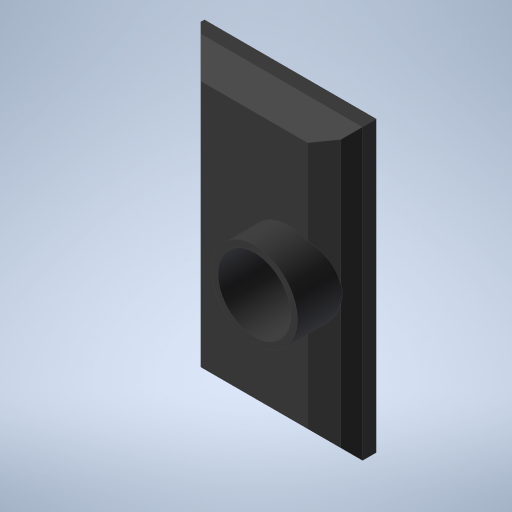
# Autodesk Inventor part: Part5
Saved by Autodesk Inventor 2024 (Build 280153000, 153)
## iProperties
Created: 2024-06-14
Part Number: Part5
Material: Generic
Document SubType Name: Sheet Metal
Designer: albah
Density: 1 g/cm^3
Sheet Metal Rule: Default_mm
Appearance: Default
Author: albah
Autodesk Inventor part; units mm, degrees
ref_plane "YZ Plane" through (0, 0, 0) normal (1, 0, 0) x (0, 1, 0)
ref_plane "XZ Plane" through (0, 0, 0) normal (0, 1, 0) x (-1, 0, 0)
ref_plane "XY Plane" through (0, 0, 0) normal (0, 0, 1) x (1, 0, 0)
sketch "Sketch1" plane through (0, 0, 0) normal (0, 0, 1) x (1, 0, 0)
  line L0 (0, 0) -> (50, 0)
  line L1 (50, 0) -> (50, -84)
  line L2 (50, -84) -> (0, -84)
  line L3 (0, -84) -> (0, 0)
  circle A0 centre (34.5628, -42) radius 12.4978
  circle A1 centre (34.5628, -42) radius 10.6396
  dimension "d0" = 50
  dimension "d1" = 84
  constraints: 8 end point, 2 centre point, 2 parallel, 1 coincident, 1 horizontal, 1 perpendicular
  measures "d0" distance of L1.end L2.end
  measures "d1" distance of L0.end L1.end
extrude "Extrusion1" add sketch "Sketch1" along normal blind 10 contours L0 L1 L2 L3
extrude "Extrusion2" add sketch "Sketch1" along normal blind 20 contours A0
chamfer "Chamfer1" distance 6 angle 45 1 edges at (50, -42, 10)
chamfer "Chamfer2" distance 4 angle 45 2 edges at (44, -67.0968, 10) (44, -16.9032, 10)
chamfer "Chamfer3" distance 9 angle 45 1 edges at (0, -42, 10)
chamfer "Chamfer4" distance 6 angle 45 2 edges at (24.5, 0, 10) (24.5, -84, 10)
equation "\"BendRadius\" = Thickness"
equation "\"BendReliefWidth\" = Thickness"
equation "\"BendReliefDepth\" = 0.5 * Thickness"
equation "\"CornerReliefSize\" = 4 * Thickness"
equation "\"MinimumRemnant\" = 2 * Thickness"
equation "\"TransitionRadius\" = BendRadius"
equation "\"JacobiRadiusSize\" = BendRadius"
equation "\"GapSize\" = Thickness"
equation "\"Thickness\" = 0.5"
body "Solid1"
